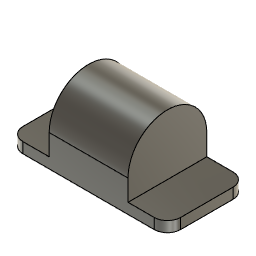
busStopPiece (Autodesk Fusion 360 archive; units mm, degrees)
design "busStop" references "TactileMapsParameters"
Autodesk Fusion 360 part; units mm, degrees
derive "ExternalDerived1" from "TactileMapsParameters v5"
sketch "Sketch1" plane through (0, 0, 0) normal (0, 0, 1) x (1, 0, 0)
  line L0 (0, 0) -> (12, 0)
  line L1 (12, 0) -> (12, 6)
  line L2 (12, 6) -> (0, 6)
  line L3 (0, 6) -> (0, 0)
  dimension "d18" = 12
  dimension "d19" = 6
  constraint horizontal L0
  constraint vertical L1
  constraint horizontal L2
  constraint vertical L3
  constraint coincident L0.start L3.end
  measures "d18" distance of L0.start L0.end
  measures "d19" distance of L0.start L2.end
extrude "Extrude1" add sketch "Sketch1" along normal blind 0.8
ref_plane "WorkPlane1" through (6, 0, 0) normal (1, 0, 0) x (0, 1, 0)
sketch "Sketch2" plane through (6, 0, 0) normal (1, 0, 0) x (0, 1, 0)
  line L0 (0, 0.8) -> (0, 2.4)
  line L1 (0, 0.8) -> (6, 0.8)
  line L2 (6, 0.8) -> (6, 2.4)
  line L3 (3, 0.8) -> (3, 2.4) construction
  arc A0 (6, 2.4) -> (0, 2.4) centre (3, 2.4) ccw
  point P0 (0, 0.8)
  point P1 (6, 0.8)
  dimension "d23" = 1.6
  dimension "d24" = 6
  dimension "d25" = 1.6
  dimension "d26" = 1.6
  constraint coincident P0 L0.start
  constraint vertical L0
  constraint perpendicular L0 L1
  constraint coincident P1 L1.end
  constraint perpendicular L1 L2
  constraint midpoint L1 L3.start
  constraint perpendicular L1 L3
  constraint coincident L3.end A0.centre
  measures "d23" distance of P0 L0.end
  measures "d24" distance of P0 P1
  measures "d25" distance of P1 L2.end
  measures "d26" distance of L3.start L3.end
extrude "Extrude2" add sketch "Sketch2" along normal mid plane 6
fillet "Fillet1" radius 1 4 edges at (0, 0, 0.4) (12, 0, 0.4) (12, 6, 0.4) (0, 6, 0.4)
equation "length_Ref = 170 mm" comment "Side lengths of base of model"
equation "baseHeight_Ref = 0.4 mm" comment "Height of the base of the model"
equation "sidewalkHeight_Ref = 3.2 mm" comment "Height of sidewalk/walking surface"
equation "sidewalkWidth_Ref = length_Ref / 3" comment "Width of the sidewalk/walking surface"
equation "orientorSize_Ref = 6 mm" comment "Side length of orientation indicator square"
equation "oritentorHeight_Ref = 2.4 mm" comment "Height of the orientation indicator"
equation "braileHeight_Ref = 0.6 mm" comment "Standard height of Braille characters"
equation "filletRadius_Ref = 0.6 mm" comment "Radius of fillets to soften edges"
equation "lineWidth_Ref = 3 mm" comment "Width of crosswalk lines"
equation "lineHeight_Ref = braileHeight_Ref / 2" comment "Height of crosswalk lines"
equation "tabWidth_Ref = length_Ref / 10" comment "Width of tabs to secure adjacent maps together"
equation "tabLength_Ref = length_Ref / 14" comment "Length of tab to secure adjacent maps together"
equation "tabHeight_Ref = sidewalkHeight_Ref / 4" comment "Height of tabs to secure adjacent maps together"
equation "clearance_Ref = 0.4 mm" comment "Clearance around parts that will fit together"
equation "featureHeight_Ref = 1.6 mm" comment "Height of features such as bus stops"
equation "pegSize_Ref = 6 mm" comment "Side length of pegs/holes to connect features to map base"
equation "pegDepth_Ref = sidewalkHeight_Ref / 4" comment "Depth of pegs/holes to connect features to map base"
equation "d18 = 2 * pegSize_Ref"
equation "d19 = pegSize_Ref"
equation "d20 = pegDepth_Ref"
equation "d22 = pegSize_Ref"
equation "d23 = featureHeight_Ref"
equation "d24 = pegSize_Ref"
equation "d25 = featureHeight_Ref"
equation "d26 = featureHeight_Ref"
equation "d27 = pegSize_Ref / 2"
